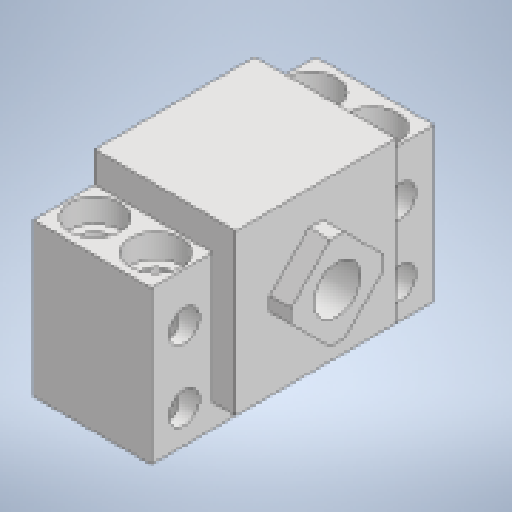
# Autodesk Inventor part: BK10_Frame
Saved by Autodesk Inventor 2023 (Build 270158000, 158)
## iProperties
Created: 2022-04-29
Part Number: BK10_Frame
Material: Generic
Document SubType Name: Modeling
Designer: plebbb
Density: 1 g/cm^3
Appearance: Default
Author: plebbb
Autodesk Inventor part; units mm, degrees
ref_plane "YZ Plane" through (0, 0, 0) normal (1, 0, 0) x (0, 1, 0)
ref_plane "XZ Plane" through (0, 0, 0) normal (0, 1, 0) x (-1, 0, 0)
ref_plane "XY Plane" through (0, 0, 0) normal (0, 0, 1) x (1, 0, 0)
sketch "Sketch1" plane through (0, 0, 0) normal (1, 0, 0) x (0, 1, 0)
  line L0 (0, 0) -> (32.5, 0)
  line L1 (32.5, 0) -> (32.5, -13)
  line L2 (32.5, -60) -> (0, -60)
  line L3 (0, -60) -> (0, 0)
  circle A0 centre (22, -53) radius 3.3
  circle A1 centre (22, -7) radius 3.3
  circle A2 centre (7, -7) radius 3.3
  circle A3 centre (7, -53) radius 3.3
  line L4 (22, -7) -> (7, -7) construction
  line L5 (7, -7) -> (7, -53) construction
  line L6 (7, -53) -> (22, -53) construction
  line L7 (22, -53) -> (22, -7) construction
  line L8 (32.5, -13) -> (39, -13)
  line L9 (39, -13) -> (39, -47)
  line L10 (39, -47) -> (32.5, -47)
  line L11 (32.5, -47) -> (32.5, -60)
  line L12 (32.5, -13) -> (32.5, -47) construction
  circle A4 centre (22, -30) radius 5
  point P0 (32.5, -30)
  dimension "d0" = 60
  dimension "d1" = 6.6
  dimension "d2" = 15
  dimension "d3" = 46
  dimension "d4" = 22
  dimension "d5" = 32.5
  dimension "d6" = 34
  dimension "d7" = 39
  dimension "d8" = 10
  constraints: 26 end point, 8 perpendicular, 6 parallel, 5 centre point, 3 coincident, 3 equal radius, 3 horizontal, 2 midpoint, 1 collinear, 1 horizontal alignment
  measures "d0" distance of L0.end L2.start
  measures "d1" diameter of A0
  measures "d2" distance of L5.end L6.end
  measures "d3" distance of L6.end L4.start
  measures "d4" horizontal distance of L0.start L4.start
  measures "d5" distance from line of L0.start L1
  measures "d6" distance of L8.end L9.end
  measures "d7" horizontal distance of L0.start L8.end
  measures "d8" diameter of A4
extrude "Extrusion1" add sketch "Sketch1" along normal blind 25
sketch "Sketch2" plane through (25, 0, 0) normal (1, 0, 0) x (0, 0, -1)
  line L0 (47, 39) -> (13, 39) projected
  line L1 (13, 39) -> (13, 5)
  line L2 (13, 5) -> (47, 5)
  line L3 (47, 5) -> (47, 39)
  circle A0 centre (30, 22) radius 5 projected
  point P0 (0, 0)
  constraints: 6 end point, 3 perpendicular, 1 vertical
extrude "Extrusion2" add sketch "Sketch2" along normal blind 5
sketch "Sketch3" plane through (30, 0, 0) normal (1, 0, 0) x (0, 0, -1)
  circle A0 centre (30, 22) radius 5 projected
  circle A1 centre (30, 22) radius 5 projected
  line L0 (20.1863, 23.5) -> (20.1863, 20.5)
  line L1 (20.1863, 20.5) -> (28.5, 12.1863)
  line L2 (28.5, 12.1863) -> (31.5, 12.1863)
  line L3 (31.5, 12.1863) -> (39.8137, 20.5)
  line L4 (39.8137, 20.5) -> (39.8137, 23.5)
  line L5 (39.8137, 23.5) -> (31.5, 31.8137)
  line L6 (31.5, 31.8137) -> (28.5, 31.8137)
  line L7 (28.5, 31.8137) -> (20.1863, 23.5)
  point P0 (0, 0)
  point P1 (30, 12.1863)
  point P2 (20.1863, 22)
  point P3 (35.6569, 27.6569)
  point P4 (24.3431, 16.3431)
  dimension "d14" = 135
  dimension "d15" = 16
  dimension "d16" = 3
  constraints: 16 end point, 4 midpoint, 3 equal length, 3 horizontal alignment, 3 parallel, 3 vertical alignment, 1 perpendicular, 1 vertical
  measures "d14" angle of L2 L1
  measures "d15" distance of point (35.657, 27.657) point (24.343, 16.343)
  measures "d16" distance of L5.end L6.end
extrude "Extrusion3" add sketch "Sketch3" along normal blind 4.5
sketch "Sketch4" plane through (0, 32.5, -47) normal (0, 1, 0) x (1, 0, 0)
  circle A0 centre (6, -40) radius 5.4
  point P0 (0, -47)
  dimension "d19" = 10.8
  dimension "d20" = 6
  dimension "d21" = 7
  constraints: 1 centre point
  measures "d19" diameter of A0
  measures "d20" horizontal distance of point (0, -47) A0.centre
  measures "d21" vertical distance of point (0, -47) A0.centre
extrude "Extrusion4" cut sketch "Sketch4" against normal blind 5
sketch "Sketch5" plane through (6, 27.5, -7) normal (0, 1, 0) x (1, 0, 0)
  circle A0 centre (0, 0) radius 3.3
  circle A1 centre (0, 0) radius 5.4 construction
  point P0 (-6, -7)
  dimension "d24" = 6.6
  constraints: 1 centre point, 1 coincident
  measures "d24" diameter of A0
extrude "Extrusion5" cut sketch "Sketch5" against normal up to surface (27.5 mm away)
pattern_linear "Rectangular Pattern1" count 2 spacing 13 along (1, 0, 0) count 2 spacing -46 along (0, 0, 1) of "Extrusion5", "Extrusion4"
body "Solid1"
